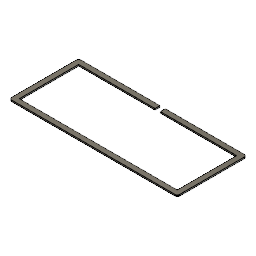
open (Autodesk Fusion 360 design; units mm, degrees)
Autodesk Fusion 360 part; units mm, degrees
sketch "Sketch1" plane through (0, 0, 0) normal (0, 1, 0) x (1, 0, 0)
  line L0 (3.5485, 0.3183) -> (3.1805, 0.4548)
  line L1 (2.825, 0.6187) -> (2.4819, 0.8103)
  line L2 (2.1553, 1.028) -> (1.8466, 1.2706)
  line L3 (324.159, 131.987) -> (324.35, 131.644)
  line L4 (324.651, 130.92) -> (324.757, 130.542)
  line L5 (314.895, 10.0748) -> (314.895, 124.375)
  line L6 (321.441, 134.13) -> (321.809, 133.993)
  line L7 (3.1805, 0.4548) -> (2.825, 0.6187)
  line L8 (321.062, 134.236) -> (321.441, 134.13)
  line L9 (324.834, 130.157) -> (324.879, 129.767)
  line L10 (323.941, 2.1346) -> (323.698, 1.8259)
  line L11 (324.834, 4.2912) -> (324.757, 3.9067)
  line L12 (3.9274, 0.2122) -> (3.5485, 0.3183)
  line L13 (2.4819, 0.8103) -> (2.1553, 1.028)
  line L14 (167.495, 124.375) -> (167.495, 134.374)
  line L15 (1.5586, 1.5379) -> (1.2912, 1.8259)
  line L16 (321.062, 0.2122) -> (320.678, 0.135)
  line L17 (321.809, 0.4548) -> (321.441, 0.3183)
  line L18 (324.757, 3.9067) -> (324.651, 3.5278)
  line L19 (324.35, 2.8043) -> (324.159, 2.4612)
  line L20 (324.757, 130.542) -> (324.834, 130.157)
  line L21 (324.514, 131.288) -> (324.651, 130.92)
  line L22 (324.159, 2.4612) -> (323.941, 2.1346)
  line L23 (157.494, 124.375) -> (10.0941, 124.375)
  line L24 (323.431, 1.5379) -> (323.143, 1.2705)
  line L25 (157.494, 134.375) -> (157.494, 124.375)
  line L26 (320.678, 134.313) -> (321.062, 134.236)
  line L27 (323.431, 132.91) -> (323.698, 132.623)
  line L28 (324.879, 129.767) -> (324.895, 129.374)
  line L29 (10.0941, 10.0748) -> (314.895, 10.0748)
  line L30 (320.288, 0.0896) -> (319.896, 0.073)
  line L31 (319.896, 0.073) -> (5.0946, 0.073)
  line L32 (5.0946, 0.073) -> (4.7019, 0.0896)
  line L33 (0.6394, 131.644) -> (0.831, 131.987)
  line L34 (1.2912, 1.8259) -> (1.0487, 2.1346)
  line L35 (167.495, 134.374) -> (319.896, 134.374)
  line L36 (0.831, 2.4612) -> (0.6394, 2.8043)
  line L37 (1.8466, 1.2706) -> (1.5586, 1.5379)
  line L38 (323.941, 132.314) -> (324.159, 131.987)
  line L39 (10.0941, 124.375) -> (10.0941, 10.0748)
  line L40 (0.4754, 3.1598) -> (0.339, 3.5278)
  line L41 (322.508, 0.8103) -> (322.165, 0.6187)
  line L42 (0.0937, 5.0739) -> (0.0951, 129.374)
  line L43 (1.8466, 133.178) -> (2.1553, 133.42)
  line L44 (0.2329, 130.542) -> (0.339, 130.92)
  line L45 (3.1805, 133.993) -> (3.5485, 134.13)
  line L46 (323.698, 132.623) -> (323.941, 132.314)
  line L47 (324.895, 129.374) -> (324.896, 5.0726)
  line L48 (320.678, 0.135) -> (320.288, 0.0896)
  line L49 (324.35, 131.644) -> (324.514, 131.288)
  line L50 (322.834, 133.42) -> (323.143, 133.178)
  line L51 (0.0951, 129.374) -> (0.1102, 129.767)
  line L52 (3.5485, 134.13) -> (3.9274, 134.236)
  line L53 (0.1102, 4.6812) -> (0.0937, 5.0739)
  line L54 (5.0946, 134.375) -> (157.494, 134.375)
  line L55 (319.896, 134.374) -> (320.288, 134.359)
  line L56 (324.896, 5.0726) -> (324.879, 4.6812)
  line L57 (0.1557, 130.157) -> (0.2329, 130.542)
  line L58 (4.7019, 134.359) -> (5.0946, 134.375)
  line L59 (322.508, 133.638) -> (322.834, 133.42)
  line L60 (4.3119, 0.135) -> (3.9274, 0.2122)
  line L61 (324.514, 3.1598) -> (324.35, 2.8043)
  line L62 (4.7019, 0.0896) -> (4.3119, 0.135)
  line L63 (324.879, 4.6812) -> (324.834, 4.2912)
  line L64 (321.441, 0.3183) -> (321.062, 0.2122)
  line L65 (321.809, 133.993) -> (322.165, 133.829)
  line L66 (0.6394, 2.8043) -> (0.4754, 3.1598)
  line L67 (0.831, 131.987) -> (1.0487, 132.314)
  line L68 (0.339, 3.5278) -> (0.2329, 3.9067)
  line L69 (2.4819, 133.638) -> (2.825, 133.829)
  line L70 (1.2912, 132.623) -> (1.5586, 132.91)
  line L71 (322.834, 1.028) -> (322.508, 0.8103)
  line L72 (320.288, 134.359) -> (320.678, 134.313)
  line L73 (1.5586, 132.91) -> (1.8466, 133.178)
  line L74 (0.2329, 3.9067) -> (0.1557, 4.2912)
  line L75 (314.895, 124.375) -> (167.495, 124.375)
  line L76 (323.143, 1.2706) -> (322.834, 1.028)
  line L77 (324.651, 3.5278) -> (324.514, 3.1598)
  line L78 (0.339, 130.92) -> (0.4754, 131.288)
  line L79 (322.165, 0.6187) -> (321.809, 0.4548)
  line L80 (4.3119, 134.313) -> (4.7019, 134.359)
  line L81 (0.1557, 4.2912) -> (0.1102, 4.6812)
  line L82 (0.1102, 129.767) -> (0.1557, 130.157)
  line L83 (3.9274, 134.236) -> (4.3119, 134.313)
  line L84 (2.825, 133.829) -> (3.1805, 133.993)
  line L85 (323.698, 1.8259) -> (323.431, 1.5379)
  line L86 (2.1553, 133.42) -> (2.4819, 133.638)
  line L87 (1.0487, 2.1346) -> (0.831, 2.4612)
  line L88 (0.4754, 131.288) -> (0.6394, 131.644)
  line L89 (1.0487, 132.314) -> (1.2912, 132.623)
  line L90 (322.165, 133.829) -> (322.508, 133.638)
  line L91 (323.143, 133.178) -> (323.431, 132.91)
extrude "Extrude1" add sketch "Sketch1" along normal blind 3
